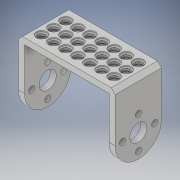
# Autodesk Inventor part: OlloToAX12
Saved by Autodesk Inventor 2017 (Build 210142000, 142)
## iProperties
Created: 2016-07-30
Part Number: OlloToAX12
Material: Generic
Document SubType Name: Modeling
Designer: Labtech
Density: 1 g/cm^3
Appearance: Default
Author: Labtech
Autodesk Inventor part; units mm, degrees
ref_plane "YZ Plane" through (0, 0, 0) normal (1, 0, 0) x (0, 1, 0)
ref_plane "XZ Plane" through (0, 0, 0) normal (0, 1, 0) x (-1, 0, 0)
sketch "Sketch2" plane through (0, 0, 0) normal (1, 0, 0) x (0, 1, 0)
  arc A0 (0, 11.5) -> (0, -11.5) centre (0, 0) ccw
  line L0 (0, 11.5) -> (0, -11.5) construction
  line L1 (0, -11.5) -> (24, -11.5)
  line L2 (24, -11.5) -> (24, 11.5)
  line L3 (24, 11.5) -> (0, 11.5)
  circle A1 centre (0, 0) radius 4.25
  circle A2 centre (0, -8) radius 1.5
  circle A3 centre (8, 0) radius 1.5
  circle A4 centre (0, 8) radius 1.5
  circle A5 centre (-8, 0) radius 1.5
  dimension "d0" = 23
  dimension "d2" = 24
  dimension "d3" = 23
  dimension "d4" = 8.5
  dimension "d5" = 3
  dimension "d6" = 8
  dimension "d9" = 360
  constraints: 8 end point, 6 centre point, 2 coincident, 2 parallel, 2 point on circle, 1 perpendicular, 1 point on line, 1 vertical, 9 other
  measures "d0" diameter of A0
  measures "d2" distance of L2.end L0.start
  measures "d3" distance of L1.end L2.end
  measures "d4" diameter of A1
  measures "d5" diameter of A2
  measures "d6" distance of A2.centre point (0, 0)
extrude "Extrusion1" add sketch "Sketch2" along normal blind 3
sketch "Sketch3" plane through (0, 0, 0) normal (-1, 0, 0) x (0, 0, 1)
  line L0 (-11.5, 24) -> (11.5, 24) projected
  line L1 (-11.5, 24) -> (11.5, 24)
  line L2 (11.5, 24) -> (11.5, 21)
  line L3 (11.5, 21) -> (-11.5, 21)
  line L4 (-11.5, 21) -> (-11.5, 24)
  point P0 (0, 0)
  dimension "d13" = 3
  constraints: 8 end point, 3 equal length, 1 perpendicular
  measures "d13" distance of L0.end L2.end
extrude "Extrusion2" add sketch "Sketch3" along normal blind 21
ref_plane "Work Plane1" through (-21, 21, -11.5) normal (-1, 0, 0) x (0, 0, 1)
mirror "Mirror1" about plane through (-21, 21, -11.5) normal (-1, 0, 0) of "Extrusion1", "Extrusion2"
sketch "Sketch4" plane through (3, 24, 11.5) normal (0, 1, 0) x (1, 0, 0)
  line L0 (-48, 23) -> (-48, 0) projected
  line L1 (-48, 11.5) -> (0, 11.5) construction
  line L2 (0, 13) -> (0, 10) projected
  circle A0 centre (-24, 11.5) radius 2.05
  point P0 (-3, 11.5)
  dimension "d16" = 4.1
  constraints: 3 midpoint, 2 end point, 1 centre point
  measures "d16" diameter of A0
extrude "Extrusion3" cut sketch "Sketch4" against normal through all
sketch "Sketch5" plane through (3, 24, 11.5) normal (0, 1, 0) x (1, 0, 0)
  circle A0 centre (-24, 11.5) radius 2.05 projected
  circle A1 centre (-24, 11.5) radius 2.6
  point P0 (-3, 11.5)
  dimension "d19" = 5.2
  constraints: 1 centre point, 1 coincident
  measures "d19" diameter of A1
extrude "Extrusion4" cut sketch "Sketch5" against normal blind 1
sketch "Sketch7" plane through (0, 21, -11.5) normal (0, -1, 0) x (1, 0, 0)
  circle A0 centre (-21, 11.5) radius 2.05 projected
  circle A1 centre (-21, 11.5) radius 2.6
  point P0 (0, 11.5)
  dimension "d22" = 5.2
  constraints: 1 centre point, 1 coincident
  measures "d22" diameter of A1
extrude "Extrusion5" cut sketch "Sketch7" against normal blind 1
chamfer "Chamfer1" distance 0.5 angle 45 1 edges at (-23.6, 22, 0)
chamfer "Chamfer2" distance 0.5 angle 45 1 edges at (-23.6, 23, 0)
pattern_linear "Rectangular Pattern1" count 2 spacing 6 along (0, 0, 1) count 2 spacing 6 along (0, 0, -1) of "Extrusion3", "Extrusion4", "Extrusion5", "Chamfer1", "Chamfer2"
pattern_linear "Rectangular Pattern2" count 4 spacing 6 along (1, 0, 0) count 4 spacing 6 along (-1, 0, 0) of "Rectangular Pattern1", "Extrusion3", "Extrusion4", "Extrusion5", "Chamfer1", "Chamfer2"
chamfer "Chamfer3" distance 2 angle 45 2 edges at (-45, 24, 0) (3, 24, 0)
body "Solid1"
